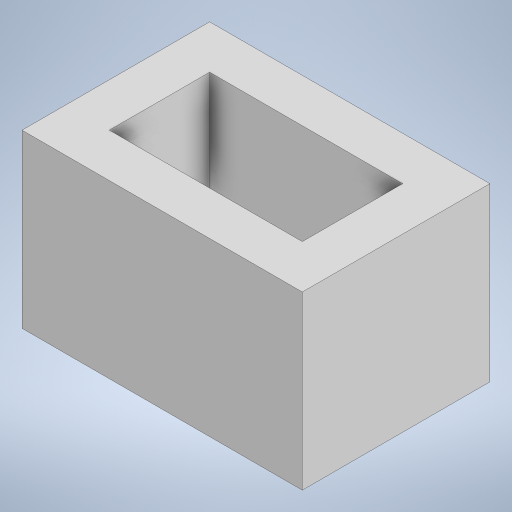
# Autodesk Inventor part: switch test v02b
Saved by Autodesk Inventor 2023.5 (Build 275446000, 446)
## iProperties
Created: 2024-08-19
Part Number: switch test v02b
Material: Generic
Document SubType Name: Modeling
Designer: Akramilab
Density: 1 g/cm^3
Appearance: Default
Author: Akramilab
Autodesk Inventor part; units mm, degrees
ref_plane "YZ Plane" through (0, 0, 0) normal (1, 0, 0) x (0, 1, 0)
ref_plane "XZ Plane" through (0, 0, 0) normal (0, 1, 0) x (-1, 0, 0)
ref_plane "XY Plane" through (0, 0, 0) normal (0, 0, 1) x (1, 0, 0)
sketch "Sketch1" plane through (0, 0, 0) normal (0, 1, 0) x (-1, 0, 0)
  line L0 (0, 0) -> (-13.27, 0)
  line L1 (-13.27, 0) -> (-13.27, 6.9)
  line L2 (-13.27, 6.9) -> (0, 6.9)
  line L3 (0, 6.9) -> (0, 0)
  line L4 (3, -3) -> (-16.27, -3)
  line L5 (-16.27, -3) -> (-16.27, 9.9)
  line L6 (-16.27, 9.9) -> (3, 9.9)
  line L7 (3, 9.9) -> (3, -3)
  point P0 (-6.635, -3)
  point P1 (-6.635, 0)
  point P2 (3, 3.45)
  dimension "d0" = 13.27
  dimension "d1" = 6.9
  dimension "d2" = 3
  dimension "d3" = 3
  dimension "d4" = 3
  dimension "d5" = 3
  constraints: 16 end point, 4 parallel, 3 midpoint, 2 horizontal, 2 perpendicular
  measures "d0" distance of L1.end L2.end
  measures "d1" distance of L0.end L1.end
  measures "d2" distance of point (-6.635, -3) point (-6.635, 0)
  measures "d3" distance between parallel lines of L6 L2
  measures "d4" distance from line of point (3, 3.45) L3
  measures "d5" distance between parallel lines of L5 L1
extrude "Extrusion1" add sketch "Sketch1" along normal blind 8.8
sketch "Sketch2" plane through (0, 0, 0) normal (0, -1, 0) x (1, 0, 0)
  line L0 (-3, 9.9) -> (16.27, 9.9) projected
  line L1 (16.27, -3) -> (-3, -3) projected
  line L2 (-3, 9.9) -> (16.27, 9.9)
  line L3 (16.27, 9.9) -> (16.27, -3)
  line L4 (16.27, -3) -> (-3, -3)
  line L5 (-3, -3) -> (-3, 9.9)
  point P0 (0, 0)
  point P1 (16.27, 9.9)
  constraints: 8 end point, 2 parallel, 1 horizontal, 1 perpendicular
extrude "Extrusion2" add sketch "Sketch2" along normal blind 3
sketch "Sketch3" plane through (0, 0, 0) normal (0, 1, 0) x (1, 0, 0)
  line L0 (0, -6.9) -> (0, 0) projected
  line L1 (13.27, -6.9) -> (0, -6.9) projected
  line L2 (0, 0) -> (8.3, 0)
  line L3 (8.3, 0) -> (8.3, -6.9)
  line L4 (8.3, -6.9) -> (0, -6.9)
  line L5 (0, -6.9) -> (0, 0)
  dimension "d10" = 8.3
  constraints: 8 end point, 2 parallel, 1 horizontal, 1 perpendicular, 1 point on line
  measures "d10" distance of L3.end L4.end
extrude "Extrusion3" cut sketch "Sketch3" against normal blind 3
equation "\"d3\" = d2"
equation "\"d5\" = d4"
body "Solid1"
